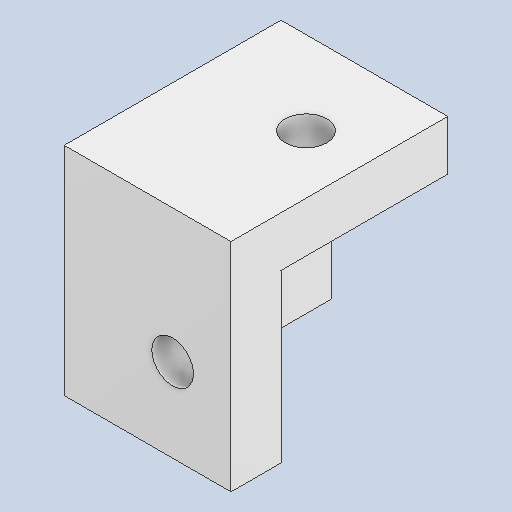
# Autodesk Inventor part: 64
Saved by Autodesk Inventor 2024.3 (Build 283343000, 343)
## iProperties
Created: 2024-09-09
Part Number: 64
Material: LCP 플라스틱
Document SubType Name: Modeling
Designer: 구지현
Density: 1.626 g/cm^3
Appearance: 매끄러움 - 흰색
Author: 구지현
Autodesk Inventor part; units mm, degrees
ref_plane "YZ Plane" through (0, 0, 0) normal (1, 0, 0) x (0, 1, 0)
ref_plane "XZ Plane" through (0, 0, 0) normal (0, 1, 0) x (-1, 0, 0)
ref_plane "XY Plane" through (0, 0, 0) normal (0, 0, 1) x (1, 0, 0)
sketch "스케치1" plane through (0, 0, 0) normal (1, 0, 0) x (0, 1, 0)
  line L0 (-5, 5) -> (5, 5)
  line L1 (5, 5) -> (5, -5)
  line L2 (5, -5) -> (-5, -5)
  line L3 (-5, -5) -> (-5, 5)
  line L4 (-5, 5) -> (5, -5) construction
  line L5 (5, 5) -> (-5, -5) construction
  point P0 (0, 0)
  dimension "d0" = 10
  dimension "d1" = 10
  constraints: 12 end point, 2 midpoint, 2 parallel, 1 horizontal, 1 perpendicular
  measures "d0" distance of L1.end L2.end
  measures "d1" distance of L0.end L1.end
extrude "돌출1" add sketch "스케치1" along normal blind 3
sketch "스케치2" plane through (0, 5, 5) normal (0, 1, 0) x (1, 0, 0)
  line L0 (0, 10) -> (0, 0) projected
  line L1 (0, 0) -> (3, 0) projected
  line L2 (3, 10) -> (3, 0) projected
  line L3 (0, 10) -> (3, 10) projected
  line L4 (0, 0) -> (10, 0)
  line L5 (10, 0) -> (10, 10)
  line L6 (10, 10) -> (0, 10)
  line L7 (0, 10) -> (0, 0)
  point P0 (0, 5)
  dimension "d4" = 10
  dimension "d5" = 10
  constraints: 8 end point, 2 parallel, 1 horizontal, 1 perpendicular
  measures "d4" distance of L6.end L5.end
  measures "d5" distance of L5.end L4.end
extrude "돌출2" add sketch "스케치2" along normal blind 3
sketch "스케치3" plane through (0, -5, 5) normal (0, 0, 1) x (1, 0, 0)
  line L0 (0, 0) -> (0, 13) projected
  line L1 (0, 0) -> (3, 0) projected
  line L2 (3, 10) -> (3, 0) projected
  line L3 (3, 10) -> (10, 10) projected
  line L4 (10, 10) -> (10, 13) projected
  line L5 (0, 13) -> (10, 13) projected
  line L6 (0, 13) -> (10, 13)
  line L7 (10, 13) -> (10, 0)
  line L8 (10, 0) -> (0, 0)
  line L9 (0, 0) -> (0, 13)
  point P0 (0, 5)
  constraints: 8 end point, 2 parallel, 1 horizontal, 1 perpendicular
extrude "돌출3" add sketch "스케치3" along normal blind 3
sketch "스케치4" plane through (3, 0, 0) normal (1, 0, 0) x (0, 0, -1)
  circle A0 centre (0, 0) radius 1.25
  dimension "d10" = 2.5
  constraints: 1 centre point, 1 coincident
  measures "d10" diameter of A0
extrude "돌출4" cut sketch "스케치4" against normal blind 3
sketch "스케치5" plane through (0, 5, 5) normal (0, -1, 0) x (1, 0, 0)
  line L0 (3, -10) -> (3, 0) projected
  line L1 (10, -10) -> (3, -10) projected
  line L2 (10, 0) -> (10, -10) projected
  line L3 (3, 0) -> (10, 0) projected
  line L4 (10, 0) -> (10, -10) projected
  line L5 (10, -5) -> (6.5, -5)
  line L6 (6.5, -5) -> (6.5, -10)
  circle A0 centre (6.5, -5) radius 1.25
  point P0 (0, -5)
  dimension "d13" = 2.5
  constraints: 4 end point, 2 midpoint, 1 centre point, 1 coincident, 1 horizontal
  measures "d13" diameter of A0
extrude "돌출5" cut sketch "스케치5" against normal blind 3 contours A0 L5 L6 | L6 L5 A0
sketch "스케치6" plane through (0, -5, 5) normal (0, 0, -1) x (-1, 0, 0)
  line L0 (-3, 10) -> (-10, 10) projected
  line L1 (-10, 0) -> (-10, 10) projected
  line L2 (-3, 0) -> (-10, 0) projected
  line L3 (-3, 10) -> (-3, 0) projected
  line L4 (-3, 0) -> (-10, 0) projected
  line L5 (-6.5, 0) -> (-6.5, 5)
  line L6 (-6.5, 5) -> (-3, 5)
  circle A0 centre (-6.5, 5) radius 1.25
  point P0 (0, 5)
  dimension "d16" = 2.5
  constraints: 4 end point, 2 midpoint, 1 centre point, 1 coincident, 1 vertical
  measures "d16" diameter of A0
extrude "돌출6" cut sketch "스케치6" against normal blind 3 contours A0 L5 L6 | L6 L5 A0
